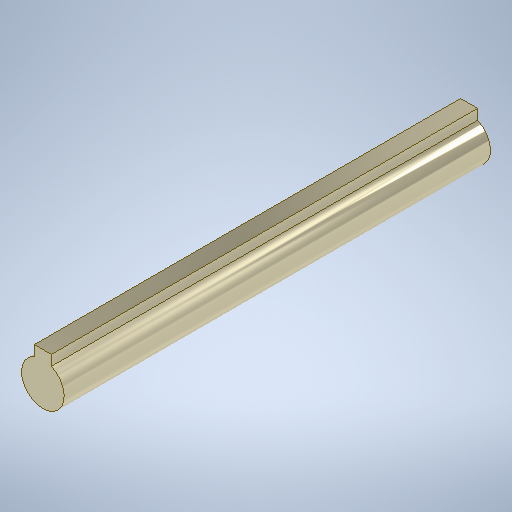
# Autodesk Inventor part: Part5
Saved by Autodesk Inventor 2025 (Build 290162000, 162)
## iProperties
Created: 2026-06-07
Part Number: Part5
Material: Generic
Document SubType Name: Modeling
Designer: user
Density: 1 g/cm^3
Appearance: Nickel
Author: user
Autodesk Inventor part; units mm, degrees
ref_plane "YZ Plane" through (0, 0, 0) normal (1, 0, 0) x (0, 1, 0)
ref_plane "XZ Plane" through (0, 0, 0) normal (0, 1, 0) x (-1, 0, 0)
ref_plane "XY Plane" through (0, 0, 0) normal (0, 0, 1) x (1, 0, 0)
sketch "Sketch1" plane through (0, 0, 0) normal (0, 0, 1) x (1, 0, 0)
  circle A0 centre (0, 0) radius 5
  line L0 (0, 0) -> (0, 7)
  line L1 (0, 7) -> (2, 7)
  line L2 (2, 7) -> (2, 0)
  line L3 (0, 7) -> (-2, 7)
  line L4 (-2, 7) -> (-2, 0)
  point P0 (2, 4.5826)
  point P1 (-2, 4.5826)
  dimension "d0" = 10
  dimension "d1" = 7
  dimension "d2" = 2
  dimension "d3" = 2
  constraints: 10 end point, 3 perpendicular, 1 centre point, 1 coincident, 1 horizontal, 1 vertical
  measures "d0" diameter of A0
  measures "d1" distance of L0.start L0.end
  measures "d2" distance of L0.end L1.end
  measures "d3" distance of L0.end L3.end
extrude "Extrusion1" add sketch "Sketch1" along normal blind 100
body "Solid1"
